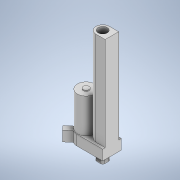
# Autodesk Inventor part: linear actuator
Saved by Autodesk Inventor 2022 (Build 260153000, 153)
## iProperties
Created: 2021-12-03
Part Number: linear actuator
Material: Generic
Document SubType Name: Modeling
Designer: efred
Density: 1 g/cm^3
Appearance: Default
Author: efred
Autodesk Inventor part; units mm, degrees
ref_plane "YZ Plane" through (0, 0, 0) normal (1, 0, 0) x (0, 1, 0)
ref_plane "XZ Plane" through (0, 0, 0) normal (0, 1, 0) x (-1, 0, 0)
ref_plane "XY Plane" through (0, 0, 0) normal (0, 0, 1) x (1, 0, 0)
sketch "Sketch1" plane through (0, 0, 0) normal (0, 1, 0) x (-1, 0, 0)
  circle A0 centre (0, 0) radius 14.75
  line L0 (-20.25, 14.75) -> (-20.25, -14.75)
  line L1 (0, 14.75) -> (-20.25, 14.75)
  line L2 (0, -14.75) -> (-20.25, -14.75)
  point P0 (14.75, 0)
  dimension "d0" = 29.5
  dimension "d1" = 35
  constraints: 6 end point, 3 point on circle, 2 tangent, 1 centre point, 1 coincident, 1 horizontal, 1 horizontal alignment, 1 parallel, 1 vertical
  measures "d0" diameter of A0
  measures "d1" distance from line of A0.start L0
extrude "Extrusion1" add sketch "Sketch1" along normal blind 204.3
sketch "Sketch2" plane through (0, 0, 0) normal (0, -1, 0) x (1, 0, 0)
  line L0 (20.25, 20.275) -> (-36.05, 20.275)
  line L1 (-55.3, 6.365) -> (-55.3, 0) construction
  line L2 (-36.05, -20.275) -> (20.25, -20.275)
  line L3 (20.25, -20.275) -> (20.25, 20.275)
  line L4 (20.25, 14.75) -> (20.25, -14.75) projected
  line L5 (0, 0) -> (18.4964, 0) construction
  circle A0 centre (-36.05, 0) radius 19.25 construction
  arc A1 (-36.05, 20.275) -> (-36.05, -20.275) centre (-36.05, 0) ccw
  dimension "d6" = 38.5
  dimension "d4" = 40.55
  dimension "d5" = 75.55
  constraints: 10 end point, 3 point on circle, 2 horizontal, 2 horizontal alignment, 2 parallel, 2 tangent, 1 centre point, 1 collinear, 1 perpendicular, 1 vertical, 4 other
  measures "d4" distance between parallel lines of L2 L0
  measures "d5" distance between parallel lines of L3 L1
extrude "Extrusion2" add sketch "Sketch2" along normal blind 22.3
sketch "Sketch3" plane through (0, 204.3, 0) normal (0, 1, 0) x (1, 0, 0)
  arc A0 (0, 14.75) -> (0, -14.75) centre (0, 0) ccw projected
  circle A1 centre (0, 0) radius 10.05
  dimension "d9" = 20.1
  constraints: 1 centre point, 1 coincident
  measures "d9" diameter of A1
extrude "Extrusion3" cut sketch "Sketch3" against normal blind 150
sketch "Sketch4" plane through (0, 0, 0) normal (0, 1, 0) x (1, 0, 0)
  circle A0 centre (-36.05, 0) radius 19.05
  arc A1 (-36.05, 20.275) -> (-36.05, -20.275) centre (-36.05, 0) ccw projected
  point P0 (0, 0)
  dimension "d12" = 38.1
  constraints: 1 centre point, 1 concentric
  measures "d12" diameter of A0
extrude "Extrusion4" add sketch "Sketch4" along normal blind 75.3
sketch "Sketch5" plane through (-36.05, 75.3, 0) normal (0, 1, 0) x (1, 0, 0)
  circle A0 centre (0, 0) radius 6.375
  circle A1 centre (0, 0) radius 19.05 projected
  point P0 (36.05, 0)
  dimension "d15" = 12.75
  constraints: 1 centre point, 1 concentric
  measures "d15" diameter of A0
extrude "Extrusion5" add sketch "Sketch5" along normal blind 2 contours A0
sketch "Sketch6" plane through (0, -22.3, 0) normal (0, -1, 0) x (1, 0, 0)
  circle A0 centre (0, 0) radius 10.05 construction
  line L0 (-8.9, -8.9) -> (8.9, -8.9)
  line L1 (8.9, -8.9) -> (8.9, 8.9)
  line L2 (8.9, 8.9) -> (-8.9, 8.9)
  line L3 (-8.9, 8.9) -> (-8.9, -8.9)
  line L4 (-8.9, -8.9) -> (8.9, 8.9) construction
  line L5 (8.9, -8.9) -> (-8.9, 8.9) construction
  arc A1 (-4.25, 8.9) -> (-8.9, 4.25) centre (-4.25, 4.25) ccw
  arc A2 (-8.9, -4.25) -> (-4.25, -8.9) centre (-4.25, -4.25) ccw
  arc A3 (4.25, -8.9) -> (8.9, -4.25) centre (4.25, -4.25) ccw
  arc A4 (8.9, 4.25) -> (4.25, 8.9) centre (4.25, 4.25) ccw
  point P0 (4.25, 8.9)
  point P1 (-4.25, -8.9)
  point P2 (8.9, -4.25)
  dimension "d18" = 17.8
  dimension "d19" = 17.8
  dimension "d22" = 360
  dimension "d24" = 8.5
  constraints: 12 end point, 8 point on circle, 4 centre point, 2 midpoint, 2 parallel, 2 point on line, 2 tangent, 1 horizontal, 1 perpendicular, 17 other
  measures "d18" distance of L0.end L1.end
  measures "d19" distance of L1.end L2.end
  measures "d24" distance of A4.end A1.start
extrude "Extrusion6" add sketch "Sketch6" along normal blind 18.8 contours A2 L3 A1 L2 A4 L1 A3 L0
fillet "Fillet1" radius 2 8 edges at (7.538, -22.3, 7.538) (8.9, -22.3, 0) (7.538, -22.3, -7.538) (0, -22.3, -8.9) (-7.538, -22.3, -7.538) (-8.9, -22.3, 0) (-7.538, -22.3, 7.538) (0, -22.3, 8.9)
sketch "Sketch7" plane through (-4.25, -41.1, 8.9) normal (0, 0, 1) x (1, 0, 0)
  circle A0 centre (4.25, 6.9) radius 3.175
  line L0 (8.5, 0) -> (0, 0) projected
  point P0 (4.25, 41.1)
  point P1 (4.25, 0)
  dimension "d28" = 6.9
  dimension "d29" = 6.35
  constraints: 1 centre point, 1 midpoint, 1 vertical alignment
  measures "d28" distance from line of A0.centre L0
  measures "d29" diameter of A0
extrude "Extrusion7" cut sketch "Sketch7" against normal through all
chamfer "Chamfer1" distance 1 angle 45 2 edges at (-3.175, -34.2, 8.9) (-3.175, -34.2, -8.9)
sketch "Sketch8" plane through (0, -22.3, 0) normal (0, -1, 0) x (1, 0, 0)
  line L0 (-50.7155, 14) -> (-50.7155, -14) construction
  arc A0 (-36.05, 20.275) -> (-36.05, -20.275) centre (-36.05, 0) ccw construction
  line L1 (-54.6626, 8.0403) -> (-46.7683, 17.2103)
  line L2 (-46.7683, 17.2103) -> (-59.6518, 28.3015)
  line L3 (-59.6518, 28.3015) -> (-67.5461, 19.1315)
  line L4 (-67.5461, 19.1315) -> (-54.6626, 8.0403)
  point P0 (0, 0)
  point P1 (-50.7155, 12.6253)
  dimension "d35" = 28
  dimension "d36" = 17
  dimension "d37" = 12.1
  constraints: 10 end point, 4 point on circle, 2 parallel, 1 midpoint, 1 perpendicular, 1 point on line, 1 vertical
  measures "d35" distance of L0.start L0.end
  measures "d36" distance between parallel lines of L1 L3
  measures "d37" distance between parallel lines of L4 L2
extrude "Extrusion8" add sketch "Sketch8" against normal up to surface (22.3 mm away)
body "Solid1"
